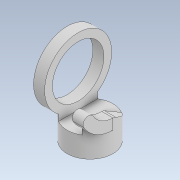
# Autodesk Inventor part: hip_front
Saved by Autodesk Inventor 2020 (Build 240168000, 168)
## iProperties
Created: 2021-01-03
Part Number: hip_front
Material: Generic
Document SubType Name: Modeling
Designer: DELL
Density: 1 g/cm^3
Appearance: Default
Author: DELL
Autodesk Inventor part; units mm, degrees
ref_plane "XZ Plane" through (0, 0, 0) normal (0, 1, 0) x (-1, 0, 0)
ref_plane "XY Plane" through (0, 0, 0) normal (0, 0, 1) x (1, 0, 0)
sketch "Sketch1" plane through (0, 0, 0) normal (0, 1, 0) x (-1, 0, 0)
  circle A0 centre (0, 0) radius 11.5 construction
  circle A1 centre (9.9593, -5.75) radius 1.65
  circle A2 centre (-9.9593, -5.75) radius 1.65
  circle A3 centre (0, 11.5) radius 1.65
  line L0 (0, 0) -> (0, 11.5) construction
  line L1 (0, 0) -> (-9.9593, -5.75) construction
  circle A4 centre (0, 0) radius 9.715 construction
  circle A5 centre (8.4134, 4.8575) radius 2
  circle A6 centre (0, -9.715) radius 2
  circle A7 centre (-8.4134, 4.8575) radius 2
  line L2 (8.4134, 4.8575) -> (0, 0) construction
  line L3 (0, 0) -> (0, -9.715) construction
  circle A8 centre (0, 0) radius 17.5 construction
  circle A9 centre (0, 0) radius 28
  circle A10 centre (9.9593, -5.75) radius 2.75
  circle A11 centre (0, 11.5) radius 2.75
  circle A12 centre (-9.9593, -5.75) radius 2.75
  line L4 (14.5, 23.9531) -> (14.5, -23.9531)
  line L5 (-14.5, 23.9531) -> (-14.5, -23.9531)
  line L6 (0, 28) -> (0, -28) construction
  line L7 (9.9593, -5.75) -> (0, 0) construction
  line L8 (-14.5, 0) -> (-28, 0)
  line L9 (-14.5, -23.9531) -> (-28, -23.9531)
  line L10 (-28, -23.9531) -> (-28, 0)
  arc A13 (-18.6667, -20.87) -> (-14.5, -19.0066) centre (-17, -19.0066) ccw
  dimension "d9" = 56
  dimension "d0" = 23
  dimension "d3" = 3.3
  dimension "d4" = 19.43
  dimension "d5" = 4
  dimension "d8" = 35
  dimension "d10" = 5.5
  dimension "d35" = 29
  dimension "d36" = 60
  dimension "d37" = 60
  dimension "d54" = 5
  constraints: 22 end point, 13 centre point, 8 coincident, 8 point on circle, 6 equal radius, 3 point on line, 2 horizontal, 2 midpoint, 2 symmetric about line, 2 vertical, 1 parallel, 1 perpendicular, 1 tangent, 12 other
  measures "d0" diameter of A0
  measures "d3" diameter of A1
  measures "d4" diameter of A4
  measures "d5" diameter of A5
  measures "d8" diameter of A8
  measures "d10" diameter of A11
  measures "d35" distance between parallel lines of L5 L4
  measures "d36" angle of L3 L7
  measures "d37" angle of L0 L2
  measures "d54" diameter of A13
extrude "Extrusion1" add sketch "Sketch1" against normal blind 25 contours A1 | A2 | A3 | A5 | A6 | A7 | A9 L4 | L4 A9 L5 | L5 L8 A9 | A9 A13 L5 | L8 L5 A13 A9 | A10 | A11 | A12
sketch "Sketch2" plane through (0, 0, 0) normal (1, 0, 0) x (0, 1, 0)
  line L0 (0, 0) -> (67.5414, 0) construction
  circle A0 centre (41, 0) radius 36
  circle A1 centre (41, 0) radius 33 construction
  line L1 (5, 0) -> (77, 0) construction
  circle A2 centre (5, 0) radius 1.75
  line L2 (23, 31.1769) -> (41, 0) construction
  circle A3 centre (41, 0) radius 41 construction
  circle A4 centre (8, 0) radius 1.75
  circle A5 centre (41, 0) radius 41
  circle A6 centre (41, 0) radius 28
  circle A7 centre (41, 0) radius 31.5
  line L3 (41, 0) -> (48.86, -0.8204) construction
  line L4 (0, -28) -> (0, 28) construction
  circle A8 centre (24.5, 28.5788) radius 1.75
  circle A9 centre (23, 31.1769) radius 1.75
  line L5 (41, 41) -> (41, -41) construction
  circle A10 centre (23, -31.1769) radius 1.75
  circle A11 centre (59, 31.1769) radius 1.75
  circle A12 centre (59, -31.1769) radius 1.75
  circle A13 centre (77, 0) radius 1.75
  circle A14 centre (23.75, 29.8779) radius 6.5
  circle A15 centre (6.5, 0) radius 6.5
  line L6 (19.641, 18.1051) -> (12.6253, 22.1557)
  line L7 (14.641, 9.4449) -> (7.6253, 13.4954)
  line L8 (41, 0) -> (5.493, 20.5) construction
  point P0 (20.5, 35.507)
  point P1 (0, 0)
  point P2 (13, 0)
  point P3 (27, 24.2487)
  dimension "d14" = 72
  dimension "d15" = 66
  dimension "d17" = 60
  dimension "d18" = 82
  dimension "d20" = 56
  dimension "d23" = 63
  dimension "d26" = 3.5
  dimension "d27" = 3.5
  dimension "d28" = 41
  dimension "d48" = 30
  dimension "d50" = 10
  constraints: 16 end point, 15 centre point, 12 point on circle, 7 coincident, 5 point on line, 4 symmetric about line, 4 tangent, 3 midpoint, 2 horizontal, 1 concentric, 1 parallel, 1 vertical, 9 other
  measures "d14" diameter of A0
  measures "d15" diameter of A1
  measures "d17" angle of L1 L2
  measures "d18" diameter of A3
  measures "d20" diameter of A6
  measures "d23" diameter of A7
  measures "d26" diameter of A4
  measures "d27" diameter of A2
  measures "d28" distance from line of L4 A6.centre
  measures "d48" angle of L0 L8
  measures "d50" distance between parallel lines of L7 L6
ref_plane "Work Plane1" through (14.5, 0, 0) normal (1, 0, 0) x (0, 1, 0)
ref_plane "Work Plane2" through (-14.5, 0, 0) normal (1, 0, 0) x (0, 1, 0)
extrude "Extrusion2" add sketch "Sketch2" against normal blind 13.5 from surface at -14.5 contours L6 A7 L7 A0 | A0 A15 A5 A14 | A0 A14 A7 L6 | L7 A7 A15 A0 | A14 A0 A9 | A0 A9 A8 A7 A14 | A15 A7 A4 A2 A0 | A0 A2 A15 | A9 A0 | A0 A9 A8 | A5 A15 A0 A10 A12 A13 A11 A14 | A2 A4 A0 | A0 A2 | A0 A14 A7 A8 A9 | A9 A8 A7 | A8 A9 | A0 A11 A13 A12 A10 A15 A7 A14 | A2 A4 A7 A15 A0 | A4 A7 A2 | A2 A4 | A11 A0 | A0 A11 | A10 A0 | A0 A10 | A13 A0 | A0 A13 | A12 A0 | A0 A12
extrude "Extrusion3" add sketch "Sketch2" along normal blind 13.5 from surface at 14.5 contours L6 A7 L7 A0 | A0 A15 A5 A14 | A0 A14 A7 L6 | L7 A7 A15 A0 | A14 A0 A9 | A0 A9 A8 A7 A14 | L6 A6 L7 A7 | A7 A14 A6 L6 | A15 A7 A4 A2 A0 | A0 A2 A15 | L7 A6 A15 A7 | A9 A0 | A0 A9 A8 | A7 A8 A14 | A2 A4 A0 | A0 A2 | A15 A7 A4 | A0 A14 A7 A8 A9 | A9 A8 A7 | A8 A9 | A7 A8 | A2 A4 A7 A15 A0 | A4 A7 A2 | A2 A4 | A4 A7
extrude "Extrusion4" add sketch "Sketch1" along normal up to surface contours A9 L4 | L5 L8 A9 round surface about axis through (0, 41, 0) along (-1, 0, 0) radius 41 far side no
sketch "Sketch3" plane through (28, 6.5, 0) normal (1, 0, 0) x (0, 0, -1)
  arc A0 (0, -6.5) -> (0, 6.5) centre (0, 0) ccw projected
  line L0 (23.9531, -6.5) -> (-23.9531, -6.5) projected
  line L1 (3.2858, 5.6084) -> (23.9531, -6.5)
  line L2 (23.9531, -6.5) -> (23.9531, 1.2246) projected
  line L3 (23.9531, -6.5) -> (23.9531, -6.5)
  dimension "d55" = 0
  constraints: 4 end point, 1 point on circle, 1 tangent, 1 vertical
  measures "d55" distance of L0.start L1.end
extrude "Extrusion5" add sketch "Sketch3" against normal up to surface (13.5 mm away)
extrude "Extrusion6" cut sketch "Sketch1" along normal through all contours L9 L10 A9
body "Solid1"
